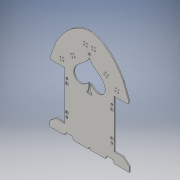
# Autodesk Inventor part: shitaita_new
Saved by Autodesk Inventor 2016 (Build 200138000, 138)
## iProperties
Created: 2016-08-31
Part Number: shitaita_new
Material: 一般
Document SubType Name: Modeling
Designer: KOTA-NPC2
Density: 1 g/cm^3
Appearance: 既定
Author: KOTA-NPC2
Autodesk Inventor part; units mm, degrees
ref_plane "YZ Plane" through (0, 0, 0) normal (1, 0, 0) x (0, 1, 0)
ref_plane "XZ Plane" through (0, 0, 0) normal (0, 1, 0) x (-1, 0, 0)
ref_plane "XY Plane" through (0, 0, 0) normal (0, 0, 1) x (1, 0, 0)
sketch "shitaita" plane through (0, 0, 0) normal (0, 0, 1) x (1, 0, 0)
  line L0 (-23.5, -2) -> (-23.5, -48)
  line L1 (23.5, -2) -> (23.5, -48)
  line L2 (-23.5, -48) -> (-32, -48)
  line L3 (-32, -48) -> (-38, -53)
  line L4 (-38, -53) -> (-38, -58)
  spline S0 degree 2 poles (-32, 15) (-18.848, 37.9416) (-1, 40) knots 0 0 0 1 1 1
  spline S1 degree 2 poles (32, 15) (18.848, 37.9416) (1, 40) knots 0 0 0 1 1 1
  line L5 (23.5, -48) -> (32, -48)
  line L6 (32, -48) -> (38, -53)
  line L7 (38, -53) -> (38, -58)
  line L8 (-1, -58) -> (0, -56)
  line L9 (1, -58) -> (0, -56)
  circle A0 centre (-21.5, -10) radius 1.05
  circle A1 centre (-21.5, -42) radius 1.05
  circle A2 centre (21.5, -10) radius 1.05
  circle A3 centre (21.5, -42) radius 1.05
  line L10 (-19.6, -21) -> (-2.4, -21) construction
  line L11 (-2.4, -21) -> (-2.4, -31) construction
  line L12 (-2.4, -31) -> (-19.6, -31) construction
  line L13 (-19.6, -31) -> (-19.6, -21) construction
  line L14 (2.4, -21) -> (19.6, -21) construction
  line L15 (19.6, -21) -> (19.6, -31) construction
  line L16 (19.6, -31) -> (2.4, -31) construction
  line L17 (2.4, -31) -> (2.4, -21) construction
  line L18 (-22.5, -13.05) -> (-20.5, -13.05)
  line L19 (-20.5, -13.05) -> (-20.5, -15.15)
  line L20 (-20.5, -15.15) -> (-22.5, -15.15)
  line L21 (-22.5, -15.15) -> (-22.5, -13.05)
  line L22 (20.5, -13.05) -> (22.5, -13.05)
  line L23 (22.5, -13.05) -> (22.5, -15.15)
  line L24 (22.5, -15.15) -> (20.5, -15.15)
  line L25 (20.5, -15.15) -> (20.5, -13.05)
  line L26 (20.5, -36.85) -> (22.5, -36.85)
  line L27 (22.5, -36.85) -> (22.5, -38.95)
  line L28 (22.5, -38.95) -> (20.5, -38.95)
  line L29 (20.5, -38.95) -> (20.5, -36.85)
  line L30 (-22.5, -36.85) -> (-20.5, -36.85)
  line L31 (-20.5, -36.85) -> (-20.5, -38.95)
  line L32 (-20.5, -38.95) -> (-22.5, -38.95)
  line L33 (-22.5, -38.95) -> (-22.5, -36.85)
  line L34 (1, -58) -> (15, -58)
  line L35 (15, -58) -> (17, -55)
  line L36 (17, -55) -> (22, -55)
  line L37 (22, -55) -> (24, -58)
  line L38 (24, -58) -> (38, -58)
  line L39 (-1, -58) -> (-15, -58)
  line L40 (-38, -58) -> (-24, -58)
  line L41 (-24, -58) -> (-22, -55)
  line L42 (-22, -55) -> (-17, -55)
  line L43 (-17, -55) -> (-15, -58)
  arc A4 (1, 40) -> (-1, 40) centre (0, 31.3293) ccw
  line L44 (-32, 15) -> (-38.5, -2)
  line L45 (-38.5, -2) -> (-23.5, -2)
  line L46 (32, 15) -> (38.5, -2)
  line L47 (38.5, -2) -> (23.5, -2)
  point P0 (0, 0)
  point P1 (-16, 34)
  point P2 (16, 34)
  dimension "d35" = 46
  dimension "d37" = 23.5
  dimension "d38" = 23.5
  dimension "d51" = 32
  dimension "d53" = 32
  dimension "d59" = 38
  dimension "d61" = 5
  dimension "d65" = 6
  dimension "d66" = 16
  dimension "d67" = 15
  dimension "d68" = 19
  dimension "d69" = 6
  dimension "d70" = 16
  dimension "d71" = 15
  dimension "d72" = 6
  dimension "d73" = 19
  dimension "d81" = 6
  dimension "d82" = 38
  dimension "d83" = 5
  dimension "d84" = 48
  dimension "d85" = 37
  dimension "d86" = 37
  dimension "d87" = 2
  dimension "d88" = 2
  dimension "d89" = 5
  dimension "d90" = 1
  dimension "d113" = 2.1
  dimension "d114" = 2.1
  dimension "d115" = 2.1
  dimension "d116" = 2.1
  dimension "d117" = 21.5
  dimension "d118" = 21.5
  dimension "d119" = 21.5
  dimension "d120" = 21.5
  dimension "d121" = 32
  dimension "d122" = 32
  dimension "d127" = 10
  dimension "d128" = 17.2
  dimension "d129" = 17.2
  dimension "d130" = 3.9
  dimension "d131" = 3.9
  dimension "d132" = 11
  dimension "d135" = 1
  dimension "d136" = 2
  dimension "d137" = 2
  dimension "d138" = 2.1
  dimension "d139" = 1
  dimension "d140" = 2
  dimension "d141" = 2
  dimension "d142" = 2.1
  dimension "d143" = 1
  dimension "d144" = 2
  dimension "d145" = 2
  dimension "d146" = 2.1
  dimension "d147" = 2
  dimension "d148" = 2.1
  dimension "d215" = 14
  dimension "d216" = 2
  dimension "d218" = 5
  dimension "d219" = 2
  dimension "d220" = 3
  dimension "d221" = 14
  dimension "d224" = 2
  dimension "d225" = 5
  constraints: 96 end point, 14 parallel, 12 horizontal, 8 perpendicular, 6 point on line, 5 centre point, 2 collinear, 2 point on circle, 2 vertical, 7 other
  measures "d35" distance of L0.start L0.end
  measures "d37" distance from line of point (0, 0) L1
  measures "d38" distance from line of L0 point (0, 0)
  measures "d51" horizontal distance of point (0, 0) L44.start
  measures "d53" horizontal distance of point (0, 0) L46.start
  measures "d59" horizontal distance of point (0, 0) L3.end
  measures "d61" vertical distance of L2.end L3.end
  measures "d65" horizontal distance of L2.end L3.end
  measures "d66" horizontal distance of L44.start point (-16, 34)
  measures "d67" horizontal distance of point (-16, 34) A4.end
  measures "d68" vertical distance of L44.start point (-16, 34)
  measures "d69" vertical distance of point (-16, 34) A4.end
  measures "d70" horizontal distance of L46.start point (16, 34)
  measures "d71" horizontal distance of A4.start point (16, 34)
  measures "d72" vertical distance of point (16, 34) A4.start
  measures "d73" vertical distance of L46.start point (16, 34)
  measures "d81" horizontal distance of L5.end L6.end
  measures "d82" horizontal distance of L6.end point (0, 0)
  measures "d83" vertical distance of L5.end L6.end
  measures "d84" vertical distance of point (0, 0) L1.end
  measures "d85" distance of L4.end L8.start
  measures "d86" distance of L7.end L9.start
  measures "d87" vertical distance of L9.start L8.end
  measures "d88" vertical distance of L8.start L8.end
  measures "d89" distance of L6.end L7.end
  measures "d90" horizontal distance of L8.end L8.start
  measures "d113" diameter of A0
  measures "d114" diameter of A1
  measures "d115" diameter of A2
  measures "d116" diameter of A3
  measures "d117" horizontal distance of point (0, 0) A0.centre
  measures "d118" horizontal distance of point (0, 0) A1.centre
  measures "d119" horizontal distance of point (0, 0) A2.centre
  measures "d120" horizontal distance of A3.centre point (0, 0)
  measures "d121" distance of A1.centre A0.centre
  measures "d122" distance of A3.centre A2.centre
  measures "d127" distance of L12.end L10.start
  measures "d128" distance of L10.start L10.end
  measures "d129" distance of L14.start L14.end
  measures "d130" distance between parallel lines of L0 L13
  measures "d131" distance between parallel lines of L1 L15
  measures "d132" distance from line of L10 A0.centre
  measures "d135" distance between parallel lines of L21 L0
  measures "d136" distance between parallel lines of L19 L21
  measures "d137" distance edge to line of A0 L18
  measures "d138" distance of L18.end L19.end
  measures "d139" distance between parallel lines of L0 L33
  measures "d140" distance of L31.end L32.end
  measures "d141" distance edge to line of A1 L32
  measures "d142" distance between parallel lines of L32 L30
  measures "d143" distance between parallel lines of L1 L23
  measures "d144" distance of L23.end L24.end
  measures "d145" distance edge to line of A2 L22
  measures "d146" distance of L24.end L22.start
  measures "d147" distance edge to line of A3 L28
  measures "d148" distance of L28.end L26.start
  measures "d215" distance of L34.end L9.start
  measures "d216" horizontal distance of L34.end L35.end
  measures "d218" distance of L35.end L36.end
  measures "d219" horizontal distance of L37.end L36.end
  measures "d220" distance from line of L36 L34.end
  measures "d221" distance of L39.end L8.start
  measures "d224" horizontal distance of L42.end L39.end
  measures "d225" distance of L41.end L42.end
sketch "肉抜き" plane through (0, 0, 0) normal (0, 0, 1) x (1, 0, 0)
  line L0 (-18, 27.0037) -> (-7, 23)
  line L1 (-7, 23) -> (-3, 23)
  line L2 (-3, 3) -> (-23.604, 3.005)
  line L3 (-23.604, 3.005) -> (-28, 15.0921)
  line L4 (-28, 15.0921) -> (-18, 27.0037)
  line L5 (3, 3) -> (23.585, 2.9479)
  line L6 (23.585, 2.9479) -> (28, 14.9831)
  line L7 (28, 14.9831) -> (18, 26.9621)
  line L8 (18, 26.9621) -> (7, 22.9899)
  line L9 (7, 22.9899) -> (3, 23.0001)
  line L10 (-3, 23) -> (-3, 3)
  line L11 (3, 23.0001) -> (3, 3)
  point P0 (0, 0)
  dimension "d91" = 20
  dimension "d92" = 3
  dimension "d93" = 24
  dimension "d95" = 15
  dimension "d96" = 3
  dimension "d97" = 160
  dimension "d98" = 120
  dimension "d99" = 110
  dimension "d100" = 3
  dimension "d101" = 15
  dimension "d102" = 3
  dimension "d103" = 160
  dimension "d104" = 24
  dimension "d105" = 20
  dimension "d107" = 120
  dimension "d108" = 110
  dimension "d159" = 6
  dimension "d171" = 25
  dimension "d172" = 25
  dimension "d173" = 11
  dimension "d174" = 11
  constraints: 24 end point, 1 horizontal, 1 parallel, 1 vertical
  measures "d91" distance of L1.end L2.start
  measures "d92" horizontal distance of point (0, 0) L2.start
  measures "d93" distance from line of L2 L0.start
  measures "d95" horizontal distance of L1.end L0.start
  measures "d96" horizontal distance of point (0, 0) L2.start
  measures "d97" angle of L1 L0
  measures "d98" angle of L3 L4
  measures "d99" angle of L2 L3
  measures "d100" horizontal distance of point (0, 0) L5.start
  measures "d101" horizontal distance of L9.end L7.end
  measures "d102" horizontal distance of point (0, 0) L5.start
  measures "d103" angle of L9 L8
  measures "d104" distance from line of L5 L7.end
  measures "d105" distance between parallel lines of L5 L9
  measures "d107" angle of L6 L7
  measures "d108" angle of L5 L6
  measures "d159" distance of L9.end L1.end
  measures "d171" distance from line of L10 L3.end
  measures "d172" distance from line of L11 L6.end
  measures "d173" horizontal distance of L0.end L0.start
  measures "d174" horizontal distance of L8.end L7.end
ref_plane "作業平面1" through (0, 0, 0.5) normal (0, 0, 1) x (1, 0, 0)
sketch "スペード" plane through (0, 0, 0.5) normal (0, 0, 1) x (1, 0, 0)
  spline S0 degree 4 poles (0, 18) (-1.4423, 13.6996) (-12.6116, 7.4671) (-21.1598, 0.3372) (-9.9497, -12.6913) (-1, -3) knots 0 0 0 0 0 0.484032 1 1 1 1 1
  spline S1 degree 4 poles (0, 18) (1.4423, 13.6996) (12.6116, 7.4671) (21.1598, 0.3372) (9.9497, -12.6913) (1, -3) knots 0 0 0 0 0 0.484032 1 1 1 1 1
  spline S2 degree 2 poles (1, -3) (-0.3472, -6.0827) (2.5, -12) knots 0 0 0 1 1 1
  spline S3 degree 2 poles (-1, -3) (0.3472, -6.0827) (-2.5, -12) knots 0 0 0 1 1 1
  line L0 (-2.5, -12) -> (2.5, -12)
  circle A0 centre (0, 21) radius 1
  point P0 (0, 0)
  point P1 (-5, 12)
  point P2 (-12, 6)
  point P3 (-15, 0)
  point P4 (5, 12)
  point P5 (12, 6)
  point P6 (15, 0)
  point P7 (-13, -6)
  point P8 (13, -6)
  point P9 (0.6, -6)
  point P10 (-0.6, -6)
  dimension "d182" = 12
  dimension "d183" = 12
  dimension "d184" = 15
  dimension "d185" = 15
  dimension "d186" = 13
  dimension "d187" = 13
  dimension "d188" = 21
  dimension "d189" = 21
  dimension "d191" = 0
  dimension "d193" = 1
  dimension "d194" = 1
  dimension "d195" = 6
  dimension "d196" = 6
  dimension "d197" = 6
  dimension "d198" = 6
  dimension "d199" = 6
  dimension "d200" = 6
  dimension "d202" = 18
  dimension "d203" = 0.6
  dimension "d204" = 2.5
  dimension "d206" = 0.6
  dimension "d207" = 2.5
  dimension "d208" = 9
  dimension "d209" = 3
  dimension "d210" = 3
  dimension "d252" = 2
  dimension "d253" = 3
  dimension "d254" = 0
  dimension "d368" = 5
  dimension "d369" = 5
  dimension "d370" = 6
  dimension "d371" = 6
  constraints: 2 end point, 1 centre point, 1 horizontal, 18 other
  measures "d182" horizontal distance of point (0, 0) point (-12, 6)
  measures "d183" horizontal distance of point (0, 0) point (12, 6)
  measures "d184" distance of point (0, 0) point (-15, 0)
  measures "d185" distance of point (0, 0) point (15, 0)
  measures "d186" horizontal distance of point (0, 0) point (-13, -6)
  measures "d187" horizontal distance of point (0, 0) point (13, -6)
  measures "d188" vertical distance of point (-1, -3) point (0, 18)
  measures "d189" vertical distance of point (1, -3) point (0, 18)
  measures "d191" horizontal distance of point (0, 0) point (0, 18)
  measures "d193" horizontal distance of point (0, 0) point (-1, -3)
  measures "d194" horizontal distance of point (0, 0) point (1, -3)
  measures "d195" vertical distance of point (12, 6) point (5, 12)
  measures "d196" vertical distance of point (-5, 12) point (-12, 6)
  measures "d197" vertical distance of point (-15, 0) point (-12, 6)
  measures "d198" vertical distance of point (15, 0) point (12, 6)
  measures "d199" vertical distance of point (-13, -6) point (-15, 0)
  measures "d200" vertical distance of point (13, -6) point (15, 0)
  measures "d202" distance of point (0, 0) point (0, 18)
  measures "d203" horizontal distance of point (0, 0) point (0.6, -6)
  measures "d204" horizontal distance of L0.end point (0, 0)
  measures "d206" horizontal distance of point (0, 0) point (-0.6, -6)
  measures "d207" horizontal distance of point (0, 0) L0.start
  measures "d208" distance from line of L0 point (-1, -3)
  measures "d209" vertical distance of point (1, -3) point (0.6, -6)
  measures "d210" vertical distance of point (-0.6, -6) point (-1, -3)
  measures "d252" diameter of A0
  measures "d253" distance of point (0, 18) A0.centre
  measures "d254" horizontal distance of point (0, 18) A0.centre
  measures "d368" horizontal distance of point (0, 0) point (-5, 12)
  measures "d369" horizontal distance of point (0, 0) point (5, 12)
  measures "d370" vertical distance of point (-5, 12) point (0, 18)
  measures "d371" vertical distance of point (5, 12) point (0, 18)
ref_plane "作業平面3" through (0, 0, 0.5) normal (0, 0, 1) x (1, 0, 0)
extrude "押し出し11" add sketch "shitaita" along normal mid plane 1
extrude "押し出し12" cut sketch "スペード" against normal blind 1
sketch "スケッチ20" plane through (0, 0, 0.5) normal (0, 0, 1) x (1, 0, 0)
  line L0 (-90, 261) -> (90, 261) construction
  line L1 (90, 261) -> (90, -99) construction
  line L2 (90, -99) -> (-90, -99) construction
  line L3 (-90, -99) -> (-90, 261) construction
  circle A0 centre (0, 21) radius 1 construction
  line L4 (-2.5, -12) -> (2.5, -12) construction
  line L5 (-20.5, -38.95) -> (-20.5, -36.85) construction
  line L6 (-20.5, -36.85) -> (-22.5, -36.85) construction
  line L7 (-22.5, -36.85) -> (-22.5, -38.95) construction
  line L8 (-22.5, -38.95) -> (-20.5, -38.95) construction
  line L9 (22.5, -38.95) -> (22.5, -36.85) construction
  line L10 (22.5, -36.85) -> (20.5, -36.85) construction
  line L11 (20.5, -36.85) -> (20.5, -38.95) construction
  line L12 (20.5, -38.95) -> (22.5, -38.95) construction
  line L13 (22.5, -15.15) -> (22.5, -13.05) construction
  line L14 (22.5, -13.05) -> (20.5, -13.05) construction
  line L15 (20.5, -13.05) -> (20.5, -15.15) construction
  line L16 (20.5, -15.15) -> (22.5, -15.15) construction
  line L17 (-20.5, -15.15) -> (-20.5, -13.05) construction
  line L18 (-20.5, -13.05) -> (-22.5, -13.05) construction
  line L19 (-22.5, -13.05) -> (-22.5, -15.15) construction
  line L20 (-22.5, -15.15) -> (-20.5, -15.15) construction
  circle A1 centre (21.5, -42) radius 1.05 construction
  circle A2 centre (21.5, -10) radius 1.05 construction
  circle A3 centre (-21.5, -42) radius 1.05 construction
  circle A4 centre (-21.5, -10) radius 1.05 construction
  line L21 (-23.5, -2) -> (-38.5, -2) construction
  line L22 (-38.5, -2) -> (-32, 15) construction
  arc A5 (1, 40) -> (-1, 40) centre (0, 31.3293) ccw construction
  line L23 (32, 15) -> (38.5, -2) construction
  line L24 (38.5, -2) -> (23.5, -2) construction
  line L25 (23.5, -2) -> (23.5, -48) construction
  line L26 (23.5, -48) -> (32, -48) construction
  line L27 (32, -48) -> (38, -53) construction
  line L28 (38, -53) -> (38, -58) construction
  line L29 (38, -58) -> (24, -58) construction
  line L30 (24, -58) -> (22, -55) construction
  line L31 (22, -55) -> (17, -55) construction
  line L32 (17, -55) -> (15, -58) construction
  line L33 (15, -58) -> (1, -58) construction
  line L34 (1, -58) -> (0, -56) construction
  line L35 (0, -56) -> (-1, -58) construction
  line L36 (-1, -58) -> (-15, -58) construction
  line L37 (-15, -58) -> (-17, -55) construction
  line L38 (-17, -55) -> (-22, -55) construction
  line L39 (-22, -55) -> (-24, -58) construction
  line L40 (-24, -58) -> (-38, -58) construction
  line L41 (-38, -58) -> (-38, -53) construction
  line L42 (-38, -53) -> (-32, -48) construction
  line L43 (-32, -48) -> (-23.5, -48) construction
  line L44 (-23.5, -48) -> (-23.5, -2) construction
  line L45 (-130.0073, -9) -> (167.0033, -9) construction
  line L46 (0, 267.6396) -> (0, -183.9131) construction
  line L47 (-132.0311, 81) -> (131.679, 81) construction
  line L48 (-84, -93) -> (84, -93) construction
  line L49 (84, -93) -> (84, 75) construction
  line L50 (84, 75) -> (-84, 75) construction
  line L51 (-84, 75) -> (-84, -93) construction
  line L52 (-84, -93) -> (84, 75) construction
  line L53 (-130.0073, 171) -> (131.679, 171) construction
  line L54 (-84, 87) -> (84, 87) construction
  line L55 (84, 87) -> (84, 255) construction
  line L56 (84, 255) -> (-84, 255) construction
  line L57 (-84, 255) -> (-84, 87) construction
  line L58 (-84, 87) -> (84, 255) construction
  line L59 (84, 87) -> (-84, 255) construction
  line L60 (15.6319, 15) -> (45.6319, 15) construction
  line L61 (28.25, 52.9329) -> (28.25, -6.076) construction
  line L62 (28.25, 15) -> (26.5135, 5.1519) construction
  line L63 (26.5135, 5.1519) -> (27.7642, 4.9314) construction
  circle A6 centre (27.7642, 4.9314) radius 0.5
  circle A7 centre (25.2628, 5.3725) radius 0.5
  line L64 (26.5135, 5.1519) -> (25.2628, 5.3725) construction
  line L65 (17.4646, 21.5) -> (33.3516, 21.5) construction
  line L66 (28.25, 15) -> (30.7613, 14.5572) construction
  line L67 (21.5, 32.1962) -> (21.5, 20) construction
  line L68 (84, 87) -> (84, 75) construction
  line L69 (21.5, 21.5) -> (16.5, 12.8397) construction
  line L70 (16.5, 12.8397) -> (17.5999, 12.2047) construction
  circle A8 centre (17.5999, 12.2047) radius 0.5
  line L71 (21.5, 21.5) -> (23.7084, 20.225) construction
  line L72 (16.5, 12.8397) -> (15.4001, 13.4747) construction
  circle A9 centre (15.4001, 13.4747) radius 0.5
  line L73 (21.5, 21.5) -> (19.2916, 22.775) construction
  line L74 (13.8265, 28.5) -> (22.8265, 28.5) construction
  line L75 (15, 34.2289) -> (15, 25.2289) construction
  line L76 (15, 28.5) -> (5.0586, 27.4194) construction
  line L77 (5.0586, 27.4194) -> (5.3341, 24.8843) construction
  circle A10 centre (5.1958, 26.1568) radius 0.5
  line L78 (15, 28.5) -> (15.2756, 25.9649) construction
  line L79 (15.2756, 25.9649) -> (5.3341, 24.8843) construction
  line L80 (5.0586, 27.4194) -> (4.783, 29.9545) construction
  circle A11 centre (4.9213, 28.682) radius 0.5
  line L81 (15, 28.5) -> (14.7244, 31.0351) construction
  line L82 (14.7244, 31.0351) -> (4.783, 29.9545) construction
  line L83 (15, 28.5) -> (84, 36) construction
  line L84 (-84, 87) -> (-84, 75) construction
  circle A12 centre (2.3962, 28.4075) radius 0.5
  circle A13 centre (2.6707, 25.8824) radius 0.5
  circle A14 centre (14.1301, 11.275) radius 0.5
  line L85 (4.9213, 28.682) -> (2.3962, 28.4075) construction
  line L86 (5.1958, 26.1568) -> (2.6707, 25.8824) construction
  line L87 (15.4001, 13.4747) -> (14.1301, 11.275) construction
  circle A15 centre (16.3299, 10.005) radius 0.5
  line L88 (17.5999, 12.2047) -> (16.3299, 10.005) construction
  circle A16 centre (27.3232, 2.43) radius 0.5
  circle A17 centre (24.8217, 2.871) radius 0.5
  line L89 (27.7642, 4.9314) -> (27.3232, 2.43) construction
  line L90 (25.2628, 5.3725) -> (24.8217, 2.871) construction
  line L91 (-28.25, 15) -> (-26.5135, 5.1519) construction
  line L92 (-26.5135, 5.1519) -> (-27.7642, 4.9314) construction
  circle A18 centre (-27.7642, 4.9314) radius 0.5
  circle A19 centre (-25.2628, 5.3725) radius 0.5
  line L93 (-26.5135, 5.1519) -> (-25.2628, 5.3725) construction
  line L94 (-28.25, 15) -> (-30.7613, 14.5572) construction
  line L95 (-21.5, 21.5) -> (-16.5, 12.8397) construction
  line L96 (-16.5, 12.8397) -> (-17.5999, 12.2047) construction
  circle A20 centre (-17.5999, 12.2047) radius 0.5
  circle A21 centre (-15.4001, 13.4747) radius 0.5
  line L97 (-16.5, 12.8397) -> (-15.4001, 13.4747) construction
  line L98 (-15, 28.5) -> (-5.0586, 27.4194) construction
  line L99 (-5.0586, 27.4194) -> (-5.3341, 24.8843) construction
  circle A22 centre (-5.1958, 26.1568) radius 0.5
  line L100 (-15, 28.5) -> (-15.2756, 25.9649) construction
  line L101 (-15.2756, 25.9649) -> (-5.3341, 24.8843) construction
  circle A23 centre (-4.9213, 28.682) radius 0.5
  line L102 (-14.7244, 31.0351) -> (-4.783, 29.9545) construction
  line L103 (-15, 28.5) -> (-14.7244, 31.0351) construction
  line L104 (-5.0586, 27.4194) -> (-4.783, 29.9545) construction
  line L105 (-15, 28.5) -> (-84, 36) construction
  circle A24 centre (-2.3962, 28.4075) radius 0.5
  circle A25 centre (-2.6707, 25.8824) radius 0.5
  circle A26 centre (-14.1301, 11.275) radius 0.5
  line L106 (-4.9213, 28.682) -> (-2.3962, 28.4075) construction
  line L107 (-5.1958, 26.1568) -> (-2.6707, 25.8824) construction
  line L108 (-15.4001, 13.4747) -> (-14.1301, 11.275) construction
  circle A27 centre (-16.3299, 10.005) radius 0.5
  line L109 (-17.5999, 12.2047) -> (-16.3299, 10.005) construction
  circle A28 centre (-27.3232, 2.43) radius 0.5
  circle A29 centre (-24.8217, 2.871) radius 0.5
  line L110 (-27.7642, 4.9314) -> (-27.3232, 2.43) construction
  line L111 (-25.2628, 5.3725) -> (-24.8217, 2.871) construction
  line L112 (-21.5, 21.5) -> (-23.7084, 20.225) construction
  line L113 (28.25, 15) -> (71.1823, 258.4812) construction
  line L114 (-28.25, 15) -> (-71.1823, 258.4812) construction
  line L115 (21.5, 21.5) -> (99.7375, 157.0113) construction
  line L116 (-21.5, 21.5) -> (-99.7375, 157.0113) construction
  point P0 (0, 0)
  point P1 (0, 261)
  point P2 (0, -9)
  point P3 (0, 171)
  point P4 (84, 171)
  dimension "d296" = 17
  dimension "d297" = 4.75
  dimension "d301" = 10
  dimension "d302" = 1.27
  dimension "d303" = 1
  dimension "d305" = 2.55
  dimension "d306" = 23.5
  dimension "d307" = 21.5
  dimension "d308" = 10
  dimension "d309" = 1.27
  dimension "d310" = 1
  dimension "d311" = 2.55
  dimension "d314" = 15
  dimension "d315" = 28.5
  dimension "d322" = 10
  dimension "d323" = 2.55
  dimension "d324" = 1
  dimension "d325" = 1.27
  dimension "d326" = 2.55
  dimension "d327" = 45
  dimension "d332" = 1
  dimension "d333" = 1
  dimension "d334" = 1
  dimension "d336" = 2.54
  dimension "d337" = 2.54
  dimension "d338" = 2.54
  dimension "d339" = 1
  dimension "d340" = 2.54
  dimension "d341" = 1
  dimension "d342" = 1
  dimension "d343" = 2.54
  dimension "d344" = 2.54
  dimension "d366" = 10
  dimension "d367" = 30
  constraints: 152 end point, 45 symmetric about line, 24 centre point, 18 coincident, 16 point on line, 15 perpendicular, 9 horizontal, 8 parallel, 5 midpoint, 4 collinear, 4 vertical, 34 other
  measures "d296" distance between parallel lines of L24 L60
  measures "d297" distance between parallel lines of L61 L25
  measures "d301" distance of L62.start L62.end
  measures "d302" distance of L62.end L63.end
  measures "d303" diameter of A6
  measures "d305" distance of L62.start L66.end
  measures "d306" distance between parallel lines of L65 L24
  measures "d307" distance from line of point (0, 0) L67
  measures "d308" distance of L69.start L69.end
  measures "d309" distance of L69.end L70.end
  measures "d310" diameter of A8
  measures "d311" distance of L69.start L71.end
  measures "d314" distance from line of point (0, 0) L75
  measures "d315" distance from line of point (0, 0) L74
  measures "d322" distance of L76.start L76.end
  measures "d323" distance of L76.end L77.end
  measures "d324" diameter of A10
  measures "d325" distance from line of L76 L86.start
  measures "d326" distance of L76.start L78.end
  measures "d327" distance from line of L45 L83.end
  measures "d332" diameter of A12
  measures "d333" diameter of A13
  measures "d334" diameter of A14
  measures "d336" distance of L85.start L85.end
  measures "d337" distance of L86.start L86.end
  measures "d338" distance of L72.end L87.end
  measures "d339" diameter of A15
  measures "d340" distance of L88.start L88.end
  measures "d341" diameter of A16
  measures "d342" diameter of A17
  measures "d343" distance of L89.start L89.end
  measures "d344" distance of L64.end L90.end
  measures "d366" angle of L46 L113
  measures "d367" angle of L46 L115
extrude "押し出し16" cut sketch "スケッチ20" against normal blind 1
chamfer "面取り1" distance 2 angle 45 2 edges at (38.5, -2, 0) (-38.5, -2, 0)
